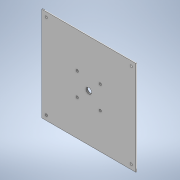
# Autodesk Inventor part: base 2
Saved by Autodesk Inventor 2022 (Build 260153000, 153)
## iProperties
Created: 2021-01-16
Part Number: base 2
Material: Generic
Document SubType Name: Modeling
Designer: chris
Density: 1 g/cm^3
Appearance: Default
Author: chris
Autodesk Inventor part; units mm, degrees
ref_plane "YZ Plane" through (0, 0, 0) normal (1, 0, 0) x (0, 1, 0)
ref_plane "XZ Plane" through (0, 0, 0) normal (0, 1, 0) x (-1, 0, 0)
ref_plane "XY Plane" through (0, 0, 0) normal (0, 0, 1) x (1, 0, 0)
sketch "Sketch1" plane through (0, 0, 0) normal (0, 0, 1) x (1, 0, 0)
  line L0 (-63.5, 63.5) -> (63.5, 63.5)
  line L1 (63.5, 63.5) -> (63.5, -63.5)
  line L2 (63.5, -63.5) -> (-63.5, -63.5)
  line L3 (-63.5, -63.5) -> (-63.5, 63.5)
  circle A0 centre (-57.15, 57.15) radius 1.524
  circle A1 centre (57.15, 57.15) radius 1.524
  line L4 (63.5, 0) -> (-63.5, 0)
  circle A2 centre (-57.15, -57.15) radius 1.524
  circle A3 centre (57.15, -57.15) radius 1.524
  point P0 (0, 0)
  point P1 (0, 63.5)
  dimension "d0" = 127
  dimension "d1" = 127
  dimension "d2" = 127
  dimension "d3" = 3.048
  dimension "d4" = 3.048
  dimension "d5" = 6.35
  dimension "d6" = 6.35
  dimension "d7" = 6.35
  dimension "d8" = 6.35
  constraints: 10 end point, 4 centre point, 3 midpoint, 2 perpendicular, 2 symmetric about line, 1 horizontal, 1 horizontal alignment, 1 vertical alignment, 2 other
  measures "d0" distance of L0.start L0.end
  measures "d1" distance of L0.end L1.end
  measures "d2" distance of L1.end L2.end
  measures "d3" diameter of A0
  measures "d4" diameter of A1
  measures "d5" distance from line of L3 A0.centre
  measures "d6" distance from line of L0 A0.centre
  measures "d7" distance from line of L0 A1.centre
  measures "d8" distance from line of L1 A1.centre
extrude "Extrusion1" add sketch "Sketch1" along normal blind 3.175
sketch "Sketch2" plane through (0, 0, 3.175) normal (0, 0, 1) x (1, 0, 0)
  circle A0 centre (0, 0) radius 3.81
  circle A1 centre (-15.494, 15.494) radius 1.524
  circle A2 centre (15.494, 15.494) radius 1.524
  circle A3 centre (-15.494, -15.494) radius 1.524
  circle A4 centre (15.494, -15.494) radius 1.524
  line L0 (-15.494, 15.494) -> (15.494, 15.494)
  line L1 (-15.494, -15.494) -> (-15.494, 15.494)
  point P0 (0, 15.494)
  point P1 (-15.494, 0)
  dimension "d11" = 7.62
  dimension "d12" = 3.048
  dimension "d13" = 3.048
  dimension "d14" = 3.048
  dimension "d15" = 3.048
  dimension "d16" = 30.988
  dimension "d21" = 30.988
  dimension "d22" = 30.988
  constraints: 5 centre point, 4 end point, 3 vertical alignment, 2 midpoint, 1 coincident, 1 horizontal, 1 horizontal alignment, 1 vertical
  measures "d11" diameter of A0
  measures "d12" diameter of A1
  measures "d13" diameter of A2
  measures "d14" diameter of A3
  measures "d15" diameter of A4
  measures "d16" distance of L0.end L0.start
  measures "d21" distance of L1.start L0.start
  measures "d22" distance of A4.centre L0.end
extrude "Extrusion2" cut sketch "Sketch2" against normal blind 25.4
fillet "Fillet1" radius 3.175 4 edges at (0, 63.5, 0) (-63.5, 0, 0) (0, -63.5, 0) (63.5, 0, 0)
sketch "Sketch4" plane through (0, 0, 0) normal (0, 0, -1) x (-1, 0, 0)
  circle A0 centre (0, 0) radius 3.81 projected
  line L0 (0, 0) -> (50.8, 0)
  line L1 (60.325, 60.325) -> (60.325, -60.325) projected
  line L2 (-60.325, 60.325) -> (60.325, 60.325) projected
  line L3 (0, 60.325) -> (60.325, 60.325)
  line L4 (63.5, 63.5) -> (63.5, -63.5) projected
  line L5 (60.325, 60.325) -> (60.325, 47.625)
  line L6 (25.4, 0) -> (25.4, 47.625)
  circle A1 centre (25.4, 47.625) radius 3.75
  circle A2 centre (50.8, 0) radius 3.75
  circle A3 centre (25.4, -47.625) radius 3.75
  line L7 (25.4, 47.625) -> (50.8, 0)
  line L8 (50.8, 0) -> (25.4, -47.625)
  line L9 (27.0544, 48.5074) -> (52.925, 0)
  line L10 (52.925, 0) -> (27.0544, -48.5074)
  line L11 (23.7456, 46.7426) -> (48.675, 0)
  line L12 (48.675, 0) -> (23.7456, -46.7426)
  circle A4 centre (15.494, 15.494) radius 1.524 projected
  line L13 (15.494, 0) -> (7.747, -13.4182)
  line L14 (7.747, -13.4182) -> (-7.747, -13.4182)
  line L15 (-7.747, -13.4182) -> (-15.494, 0)
  line L16 (-15.494, 0) -> (-7.747, 13.4182)
  line L17 (-7.747, 13.4182) -> (7.747, 13.4182)
  line L18 (7.747, 13.4182) -> (15.494, 0)
  line L19 (0, 60.325) -> (0, 13.4182)
  line L20 (0, 0) -> (-50.8, 0)
  line L21 (-25.4, 0) -> (-25.4, 47.625)
  circle A5 centre (-25.4, 47.625) radius 3.75
  circle A6 centre (-50.8, 0) radius 3.75
  circle A7 centre (-25.4, -47.625) radius 3.75
  line L22 (-25.4, 47.625) -> (-50.8, 0)
  line L23 (-50.8, 0) -> (-25.4, -47.625)
  line L24 (-27.0544, 48.5074) -> (-52.925, 0)
  line L25 (-52.925, 0) -> (-27.0544, -48.5074)
  line L26 (-23.7456, 46.7426) -> (-48.675, 0)
  line L27 (-48.675, 0) -> (-23.7456, -46.7426)
  circle A8 centre (-15.494, 15.494) radius 1.524
  point P0 (-25.4, 43.875)
  point P1 (-28.5827, 45.6418)
  point P2 (-50.9261, 3.7479)
  point P3 (-50.9261, -3.7479)
  point P4 (-28.5827, -45.6418)
  point P5 (-25.2739, -43.8771)
  point P6 (-47.6173, -1.9832)
  point P7 (-47.6173, 1.9832)
  point P8 (-25.4, 43.6406)
  point P9 (50.9261, 3.7479)
  point P10 (28.5827, 45.6418)
  point P11 (25.4, 43.875)
  point P12 (25.4, 43.6406)
  point P13 (47.6173, 1.9832)
  point P14 (47.6173, -1.9832)
  point P15 (25.2739, -43.8771)
  point P16 (28.5827, -45.6418)
  point P17 (50.9261, -3.7479)
  dimension "d24" = 50.8
  dimension "d25" = 12.7
  dimension "d26" = 7.5
  dimension "d27" = 7.5
  dimension "d28" = 1.875
  dimension "d29" = 1.875
  constraints: 50 end point, 14 symmetric about line, 7 centre point, 5 coincident, 3 midpoint, 2 perpendicular, 2 point on line, 1 horizontal alignment, 1 vertical, 20 other
  measures "d24" distance of L0.start L0.end
  measures "d25" distance of L1.start L5.end
  measures "d26" diameter of A1
  measures "d27" diameter of A2
  measures "d28" distance between parallel lines of L7 L9
  measures "d29" distance between parallel lines of L7 L11
extrude "Extrusion3" cut sketch "Sketch4" against normal blind 1 contours L0 L13 L14 L15 L20 A0 | A0 L20 L16 L17 L18 L0 | A2 L11 L0 | L0 L12 A2 | L6 A1 L7 A2 L11 | A6 L27 L20 | L20 L26 A6 | L26 A6 L22 A5 L21 | L11 A2 L7 L0 | L0 L8 A2 L12 | A2 L8 A3 L12 | A1 L7 L6 | L6 L7 A1 | L27 A6 L23 L20 | L20 L22 A6 L26 | L27 A7 L23 A6 | A5 L22 L21 | L21 L22 A5 | L7 A2 L9 L10 L8 | L7 A1 L9 A2 | A2 L10 A3 L8 | A3 | L23 A6 L25 L24 L22 | A6 L24 A5 L22 | L23 A7 L25 A6 | A7 | A2 L10 L9 | L24 L25 A6
sketch "Sketch5" plane through (0, 0, 0) normal (0, 0, -1) x (-1, 0, 0)
  line L0 (-7.747, 13.4182) -> (7.747, 13.4182) projected
  line L1 (7.747, 13.4182) -> (-7.747, 13.4182)
  point P0 (0, 0)
  constraints: 2 end point, 1 horizontal
body "Solid1"
